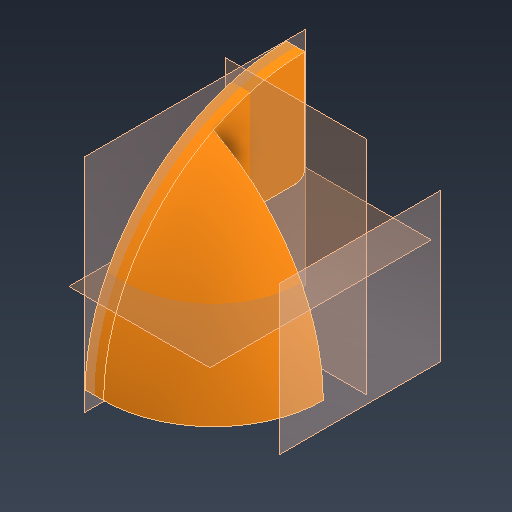
# Autodesk Inventor part: Уголок_передней_крышки_2.0
Saved by Autodesk Inventor 2023.2 (Build 272271030, 271C)
## iProperties
Created: 2025-10-06
Part Number: Уголок_передней_крышки_2.0
Material: Типовые
Document SubType Name: Modeling
Designer: Олег Коноваленко
Density: 1 g/cm^3
Appearance: Оранжевый
Author: Олег Коноваленко
Autodesk Inventor part; units mm, degrees
sketch "Эскиз1" plane through (0, 0, 0) normal (1, 0, 0) x (0, 1, 0)
  line L0 (-50, 80) -> (-50, 0)
  line L1 (-50, 0) -> (0, 0)
  line L2 (0, 0) -> (0, -30)
  line L3 (0, -30) -> (20, -30)
  line L4 (20, -30) -> (20, -45)
  line L5 (20, -45) -> (60, -45)
  line L6 (60, -45) -> (60, -30)
  arc A0 (60, -30) -> (-50, 80) centre (-50, -30) ccw
  line L7 (20, -30) -> (60, -30)
  dimension "d1" = 50
  dimension "d2" = 80
  dimension "d5" = 30
  dimension "d6" = 20
  dimension "d7" = 15
  dimension "d8" = 40
  constraints: 16 end point, 4 horizontal, 3 vertical, 2 point on circle, 1 centre point, 1 coincident, 1 line through centre, 1 parallel, 1 perpendicular
  measures "d1" distance of L0.end L1.end
  measures "d2" distance of L0.start L0.end
  measures "d5" distance of L1.end L2.end
  measures "d6" distance of L2.end L3.end
  measures "d7" distance of L3.end L4.end
  measures "d8" distance of L4.end L5.end
extrude "Выдавливание1" add sketch "Эскиз1" along normal mid plane 10 contours A0 L7 L3 L2 L1 L0
fillet "Сопряжение1" radius 5 2 edges at (0, 0, 0) (0, 0, -30)
sketch "Эскиз4" plane through (5, 0, 0) normal (1, 0, 0) x (0, 0, -1)
  arc A0 (30, 60) -> (-80, -50) centre (30, -50) ccw
  line L0 (-80, -50) -> (-50, -50)
  line L1 (-80, -50) -> (0, -50)
  arc A1 (-20, 12.44998) -> (-50, -50) centre (30, -50) ccw
  line L2 (-20, 12.44998) -> (-60.553851, 12.44998)
  line L3 (-20, -37.5) -> (-20, -62.5)
  line L4 (-20, 12.44998) -> (-20, 47.97959)
  point P0 (0, 0)
  point P1 (-20, -50)
  dimension "d16" = 30
  dimension "d19" = 25
  dimension "d20" = 30
  constraints: 8 end point, 4 point on circle, 3 point on line, 1 centre point, 1 concentric, 1 horizontal, 1 midpoint, 1 perpendicular, 1 vertical
  measures "d16" distance of L0.start L0.end
  measures "d19" distance of L3.start L3.end
  measures "d20" distance from line of L3 L0.end
sketch "Эскиз4 outline for Вращение2" plane through (5, 0, 0) normal (1, 0, 0) x (0, 0, -1)
  arc A0 (-50, -50) -> (-20, 12.44998) centre (30, -50) cw
  line L0 (-20, 12.44998) -> (-20, 47.97959)
  arc A1 (-20, 47.97959) -> (-80, -50) centre (30, -50) ccw
  line L1 (-80, -50) -> (-50, -50)
revolve "Вращение2" add sketch "Эскиз4 outline for Вращение2" angle 90 about axis through (5, -37.5, 20) along (0, 1, 0)
ref_plane "РабПлоскость1" through (35, -50, -45) normal (0, 0, 1) x (1, 0, 0)
ref_plane "РабПлоскость2" through (-5, 20, -30) normal (0, 0, 1) x (1, 0, 0)
sketch "Эскиз24" plane through (5, 60, -30) normal (0, 0, -1) x (-1, 0, 0)
  arc A0 (-20, 0) -> (-60, -40) centre (-20, -40) ccw
  line L0 (10, 0) -> (0, 0) projected
  line L1 (0, 0) -> (-20, 0)
  line L2 (-60, -40) -> (-60, -110)
  line L3 (-60, -110) -> (0, -110)
  line L4 (0, -55) -> (0, 0) projected
  line L5 (0, -110) -> (0, 0)
  constraints: 8 end point, 2 collinear, 2 point on circle, 1 centre point, 1 horizontal, 1 tangent, 1 vertical, 4 other
sketch "Эскиз18" plane through (5, 12.44998, 20) normal (0, 0, -1) x (-1, 0, 0)
  arc A0 (0, 35.52961) -> (-60, -62.44998) centre (50, -62.44998) ccw
  line L0 (-60, -62.44998) -> (-30, -62.44998)
  arc A1 (0, 0) -> (-30, -62.44998) centre (50, -62.44998) ccw
  line L1 (0, 35.52961) -> (0, 0)
  point P0 (5, -12.44998)
sketch "Эскиз19" plane through (5, 0, 0) normal (1, 0, 0) x (0, 0, -1)
  arc A0 (30, 60) -> (-20, 47.97959) centre (30, -50) ccw
  point P0 (0, 0)
ref_plane "РабПлоскость3" through (75, 0, 0) normal (1, 0, 0) x (0, 0, -1)
sketch "Эскиз23" plane through (75, 0, 0) normal (1, 0, 0) x (0, 0, -1)
  line L0 (40, -50) -> (-60, -50)
  point P0 (0, 0)
  point P1 (-20, -50)
  dimension "d111" = 100
  dimension "d112" = 40
  constraints: 2 end point, 1 horizontal, 1 point on line
  measures "d111" distance of L0.start L0.end
  measures "d112" distance of L0.end point (-20, -50)
sketch "Эскиз16" plane through (-5, 5, -30) normal (0, 0, -1) x (-1, 0, 0)
  line L0 (0, 0) -> (-10, 0)
  line L1 (0, 55) -> (0, 0)
  line L2 (0, 55) -> (-10, 55)
  line L3 (-10, 0) -> (-10, 18.536525)
  line L4 (-10, 55) -> (-30, 55)
  arc A0 (-30, 55) -> (-70, 15) centre (-30, 15) ccw
  line L5 (-70, 15) -> (-70, -55)
  line L6 (-70, -55) -> (-10, -55)
  line L7 (-10, -55) -> (-10, 0)
  point P0 (-5, -5)
sketch "Эскиз25" plane through (-5, -50, 0) normal (0, -1, 0) x (1, 0, 0)
  line L0 (0, -30) -> (0, -45) projected
  line L1 (0, -45) -> (42, -45)
  line L2 (42, -45) -> (42, 51)
  line L3 (42, 51) -> (0, 51)
  line L4 (0, 51) -> (0, -45)
  point P0 (5, 0)
  dimension "d124" = 42
  dimension "d125" = 96
  constraints: 8 end point, 2 parallel, 1 horizontal, 1 perpendicular
  measures "d124" distance of L2.end L3.end
  measures "d125" distance of L3.end L0.end
sketch "Эскиз26" plane through (-5, 0, 0) normal (-1, 0, 0) x (0, 0, 1)
  line L0 (-36.339746, 50) -> (-36.339746, 30)
  line L1 (-45, 45) -> (-36.339746, 50)
  line L2 (-36.339746, 30) -> (-45, 35)
  line L3 (-45, 20) -> (-45, 60)
  circle A0 centre (15, -35) radius 5
  point P0 (0, 0)
sketch "Эскиз27" plane through (-5, 5, -45) normal (0, 0, -1) x (-1, 0, 0)
  line L0 (-62.5, -48) -> (-60, -55) projected
  line L1 (-47.5, -48) -> (-62.5, -48) projected
  line L2 (-50, -55) -> (-47.5, -48) projected
  line L3 (-70, -55) -> (0, -55) projected
  point P0 (-5, -5)
